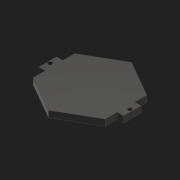
# Autodesk Inventor part: TARM16
Saved by Autodesk Inventor 2017 (Build 210142000, 142)
## iProperties
Created: 2019-07-18
Part Number: TARM16
Material: ABS Plastic
Document SubType Name: Modeling
Designer: Dell
Density: 1.06 g/cm^3
Appearance: Smooth - Black
Author: Dell
Autodesk Inventor part; units mm, degrees
ref_plane "YZ Plane" through (0, 0, 0) normal (1, 0, 0) x (0, 1, 0)
ref_plane "XZ Plane" through (0, 0, 0) normal (0, 1, 0) x (-1, 0, 0)
ref_plane "XY Plane" through (0, 0, 0) normal (0, 0, 1) x (1, 0, 0)
sketch "Sketch1" plane through (0, 0, 0) normal (0, 0, 1) x (1, 0, 0)
  line L0 (0, 66.7376) -> (57.7965, 33.3688)
  line L1 (57.7965, 33.3688) -> (57.7965, -33.3688)
  line L2 (57.7965, -33.3688) -> (0, -66.7376)
  line L3 (0, -66.7376) -> (-57.7965, -33.3688)
  line L4 (-57.7965, -33.3688) -> (-57.7965, 33.3688)
  line L5 (-57.7965, 33.3688) -> (0, 66.7376)
  line L6 (-57.7965, 15) -> (-67.7965, 15)
  line L7 (-67.7965, 15) -> (-67.7965, -15)
  line L8 (-67.7965, -15) -> (-57.7965, -15)
  line L9 (-57.7965, -15) -> (-57.7965, 15)
  line L10 (57.7965, 15) -> (67.7965, 15)
  line L11 (67.7965, 15) -> (67.7965, -15)
  line L12 (67.7965, -15) -> (57.7965, -15)
  line L13 (57.7965, -15) -> (57.7965, 15)
  circle A0 centre (-62.7965, 0) radius 3
  circle A1 centre (62.7965, 0) radius 3
  point P0 (0, 0)
  point P1 (0, 0)
  point P2 (-57.7965, 0)
  point P3 (57.7965, 0)
  point P4 (62.7965, 15)
  point P5 (-62.7965, 15)
  dimension "d0" = 10
  dimension "d1" = 30
  dimension "d2" = 30
  dimension "d3" = 10
  dimension "d4" = 133.4752
  dimension "d5" = 6
  dimension "d6" = 6
  constraints: 28 end point, 6 midpoint, 4 parallel, 3 vertical alignment, 2 centre point, 2 horizontal, 2 horizontal alignment, 2 perpendicular, 2 point on line, 1 coincident, 13 other
  measures "d0" distance of L6.start L6.end
  measures "d1" distance of L6.end L7.end
  measures "d2" distance of L10.end L11.end
  measures "d3" distance of L10.start L10.end
  measures "d4" distance of L2.end L0.start
  measures "d5" diameter of A0
  measures "d6" diameter of A1
extrude "Extrusion1" add sketch "Sketch1" along normal blind 10
sketch "Sketch2" plane through (0, 0, 10) normal (0, 0, 1) x (1, 0, 0)
  circle A0 centre (62.7965, 0) radius 3 projected
  circle A1 centre (-62.7965, 0) radius 3 projected
  line L0 (-57.7965, 15) -> (-67.7965, 15) projected
  line L1 (-67.7965, 15) -> (-67.7965, -15) projected
  line L2 (-67.7965, -15) -> (-57.7965, -15) projected
  line L3 (-57.7965, -15) -> (-57.7965, -33.3688) projected
  line L4 (-57.7965, -33.3688) -> (0, -66.7376) projected
  line L5 (0, -66.7376) -> (57.7965, -33.3688) projected
  line L6 (57.7965, -33.3688) -> (57.7965, -15) projected
  line L7 (57.7965, -15) -> (67.7965, -15) projected
  line L8 (67.7965, -15) -> (67.7965, 15) projected
  line L9 (67.7965, 15) -> (57.7965, 15) projected
  line L10 (57.7965, 15) -> (57.7965, 33.3688) projected
  line L11 (57.7965, 33.3688) -> (0, 66.7376) projected
  line L12 (0, 66.7376) -> (-57.7965, 33.3688) projected
  line L13 (-57.7965, 33.3688) -> (-57.7965, 15) projected
  line L14 (-56.7965, 32.7915) -> (0, 65.5829)
  line L15 (0, 65.5829) -> (56.7965, 32.7915)
  line L16 (56.7965, 32.7915) -> (56.7965, 14)
  line L17 (56.7965, 14) -> (66.7965, 14)
  line L18 (66.7965, 14) -> (66.7965, -14)
  line L19 (66.7965, -14) -> (56.7965, -14)
  line L20 (56.7965, -14) -> (56.7965, -32.7915)
  line L21 (56.7965, -32.7915) -> (0, -65.5829)
  line L22 (0, -65.5829) -> (-56.7965, -32.7915)
  line L23 (-56.7965, -32.7915) -> (-56.7965, -14)
  line L24 (-56.7965, -14) -> (-66.7965, -14)
  line L25 (-66.7965, -14) -> (-66.7965, 14)
  line L26 (-66.7965, 14) -> (-56.7965, 14)
  line L27 (-56.7965, 14) -> (-56.7965, 32.7915)
  point P0 (0, 0)
  dimension "d9" = 1
  constraints: 28 end point, 13 other
  measures "d9" distance between parallel lines of L12 L14
extrude "Extrusion2" cut sketch "Sketch2" against normal through all contours L13 L12 L11 L10 L9 L8 L7 L6 L5 L4 L3 L2 L1 L0
body "Solid1"
